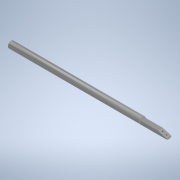
# Autodesk Inventor part: rat_headbarAngled
Saved by Autodesk Inventor 2021 (Build 250183000, 183)
## iProperties
Created: 2016-02-18
Part Number: rat_headbarAngled
Material: Stainless Steel
Document SubType Name: Modeling
Designer: Ariel
Density: 8 g/cm^3
Appearance: Aluminum - Polished
Author: Ariel
Autodesk Inventor part; units mm, degrees
ref_plane "YZ Plane" through (0, 0, 0) normal (1, 0, 0) x (0, 1, 0)
ref_plane "XZ Plane" through (0, 0, 0) normal (0, 1, 0) x (-1, 0, 0)
ref_plane "XY Plane" through (0, 0, 0) normal (0, 0, 1) x (1, 0, 0)
sketch "Sketch1" plane through (0, 0, 0) normal (1, 0, 0) x (0, 1, 0)
  circle A0 centre (0, 0) radius 6.35
  dimension "d159" = 12.7
  constraints: 1 centre point, 1 coincident
  measures "d159" diameter of A0
extrude "Extrusion1" add sketch "Sketch1" against normal blind 304.8
sketch "Sketch2" plane through (0, 0, 0) normal (1, 0, 0) x (0, 0, -1)
  arc A0 (5.9242, 2.286) -> (-5.9242, 2.286) centre (0, 0) ccw
  circle A1 centre (0, 0) radius 6.35 projected
  line L0 (-5.9242, 2.286) -> (5.9242, 2.286)
  dimension "d111" = 4.064
  constraints: 4 point on circle, 3 end point, 1 centre point, 1 coincident, 1 horizontal
  measures "d111" distance edge to line of A0 L0
extrude "Extrusion2" cut sketch "Sketch2" against normal blind 50.8 contours L0 A0
sketch "Sketch5" plane through (0, 2.286, 5.9242) normal (0, 1, 0) x (1, 0, 0)
  line L0 (0, 5.9242) -> (0, 10.7502)
  line L1 (0, 11.8485) -> (0, 0) projected
  line L2 (0, 10.7502) -> (-50.8, 10.7502)
  line L3 (-50.8, 11.8485) -> (-50.8, 0) projected
  line L4 (0, 5.9242) -> (0, 1.0982)
  line L5 (0, 1.0982) -> (-50.8, 1.0982)
  line L6 (-50.8, 1.0982) -> (-50.8, -4.826)
  line L7 (-50.8, -4.826) -> (10.2611, -4.826)
  line L8 (10.2611, -4.826) -> (0, 1.0982)
  line L9 (-50.8, 10.7502) -> (-50.8, 16.6745)
  line L10 (-50.8, 16.6745) -> (10.2611, 16.6745)
  line L11 (0, 10.7502) -> (10.2611, 16.6745)
  line L12 (-50.8, 11.8485) -> (0, 11.8485) projected
  dimension "d20" = 4.826
  dimension "d21" = 4.826
  dimension "d160" = 4.826
  constraints: 20 end point, 4 point on line, 3 equal length, 3 horizontal, 2 vertical, 1 perpendicular
  measures "d20" distance of L0.start L0.end
  measures "d21" distance of L0.start L4.end
  measures "d160" distance between parallel lines of L10 L12
extrude "Extrusion3" cut sketch "Sketch5" against normal blind 25.4 contours L2 L3 L12 L1 | L1 L12 L9 L10 L11 | L8 L7 L6 L3 L5
sketch "Sketch18" plane through (-50.8, 2.286, 4.826) normal (0, 0, 1) x (1, 0, 0)
  line L0 (34.4586, 0) -> (50.8, -4.6858)
  line L1 (0, 0) -> (50.8, 0) projected
  line L2 (34.4586, 0) -> (50.8, 0)
  line L3 (50.8, 0) -> (50.8, -4.6858)
  dimension "d144" = 17
  dimension "d161" = 74
  constraints: 6 end point, 1 collinear, 1 perpendicular
  measures "d144" distance of L0.start L0.end
  measures "d161" angle of L0 L3
extrude "Extrusion9" cut sketch "Sketch18" against normal blind 25.4
sketch "Sketch19" plane through (-16.3414, 2.286, 4.826) normal (0.2756374, 0.9612617, 0) x (0.9612617, -0.2756374, 0)
  circle A0 centre (12.4695, 4.826) radius 1.5875
  circle A1 centre (4.532, 4.826) radius 1.5875
  line L0 (14.057, 4.826) -> (17, 4.826)
  line L1 (17, 9.652) -> (17, 0) projected
  line L2 (14.057, 4.826) -> (4.532, 4.826) construction
  dimension "d148" = 3.175
  dimension "d149" = 3.175
  dimension "d151" = 7.9375
  dimension "d162" = 2.943
  constraints: 4 end point, 2 horizontal, 1 centre point, 1 horizontal alignment, 1 midpoint, 1 perpendicular, 2 other
  measures "d149" diameter of A1
  measures "d151" distance of L2.end point (12.47, 4.826)
  measures "d162" distance of L0.start L0.end
hole "Hole9" at (-11.985, 1.0368, 0) at (-4.355, -1.1511, 0) direction (-0.2756374, -0.9612617, 0) diameter 2.4867 end through all thread size "5-40 UNC" class "2B" standard "ANSI Unified Screw Threads"
equation "\"d160\" = d20"
body "Solid1"
